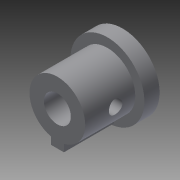
# Autodesk Inventor part: dc_to_omni_coupler_small
Saved by Autodesk Inventor 2015 (Build 190159000, 159)
## iProperties
Created: 2017-12-15
Part Number: dc_to_omni_coupler_small
Material: Generic
Document SubType Name: Modeling
Designer: Anshul
Density: 1 g/cm^3
Appearance: Default
Author: Anshul
Autodesk Inventor part; units mm, degrees
ref_plane "YZ Plane" through (0, 0, 0) normal (1, 0, 0) x (0, 1, 0)
ref_plane "XZ Plane" through (0, 0, 0) normal (0, 1, 0) x (-1, 0, 0)
sketch "Sketch1" plane through (0, 0, 0) normal (0, 1, 0) x (-1, 0, 0)
  line L0 (0, 0) -> (0, -7)
  circle A0 centre (0, -7) radius 1.55
  line L1 (3.1, 0) -> (6.4, 0)
  circle A1 centre (0, -7) radius 4
  line L2 (0, -11) -> (0, -15)
  line L3 (3.1, -15) -> (3.1, 0)
  line L4 (6.4, 0) -> (6.4, -11.5)
  line L5 (6.35, -15) -> (3.1, -15)
  line L6 (3.1, -15) -> (8.5, -15)
  line L7 (8.5, -15) -> (8.5, -11.5)
  line L8 (8.5, -11.5) -> (6.4, -11.5)
  line L9 (6.4, 0) -> (7.9, 0)
  line L10 (7.9, 0) -> (7.9, -11.5)
  line L11 (6.4, 0) -> (4.9, 0)
  line L12 (4.9, 0) -> (4.9, -11.5)
  line L13 (4.9, -11.5) -> (6.4, -11.5)
  dimension "d4" = 8
  dimension "d0" = 7
  dimension "d1" = 3.1
  dimension "d2" = 6.4
  dimension "d3" = 3.1
  dimension "d5" = 4
  dimension "d6" = 8.5
  dimension "d7" = 3.5
  dimension "d18" = 1.5
  dimension "d19" = 1.5
  constraints: 28 end point, 5 perpendicular, 3 point on line, 2 coincident, 2 horizontal, 2 parallel, 2 vertical, 1 centre point, 1 vertical alignment, 2 other
  measures "d0" distance of L0.start L0.end
  measures "d1" diameter of A0
  measures "d2" distance of L0.start L1.end
  measures "d3" distance of L1.start L0.start
  measures "d5" distance of L2.start L2.end
  measures "d6" distance of L2.end L6.end
  measures "d7" distance of L6.end L7.end
  measures "d18" distance of L1.end L9.end
  measures "d19" distance of L1.end L11.end
revolve "Revolution1" add sketch "Sketch1" angle 360 about axis through (0, 0, 0) along (0, 0, -1) picked at (3.2637, -7.5872) contours L3 L1 L12 L13 L8 L7 L6 L5 A1 | A1 L3 | L1 L4 L13 L12
ref_plane "Work Plane1" through (-6.4, 0, 0) normal (-1, 0, 0) x (0, -1, 0)
sketch "Sketch2" plane through (-6.4, 0, 0) normal (-1, 0, 0) x (0, -1, 0)
  line L0 (0, 0) -> (0, -7)
  circle A0 centre (0, -7) radius 1.55
  circle A1 centre (0, -7) radius 4
  dimension "d11" = 7
  dimension "d12" = 3.1
  dimension "d13" = 8
  constraints: 2 centre point, 2 coincident, 2 end point, 1 vertical
  measures "d11" distance of L0.start L0.end
  measures "d12" diameter of A0
  measures "d13" diameter of A1
extrude "Extrusion2" cut sketch "Sketch2" against normal blind 30 contours A0
extrude "Extrusion3" cut sketch "Sketch2" against normal blind 3
sketch "Sketch3" plane through (0, 0, 0) normal (0, 0, 1) x (1, 0, 0)
  circle A0 centre (0, 0) radius 3.1 projected
  line L0 (0, -3.1) -> (0, -6.4)
  circle A1 centre (0, 0) radius 6.4 projected
  line L1 (0, -6.4) -> (0, -7.9)
  line L2 (0, -6.4) -> (0, -4.9)
  line L3 (0, -4.9) -> (-1.5, -4.9)
  line L4 (-1.5, -4.9) -> (-1.5, -7.9)
  line L5 (-1.5, -7.9) -> (0, -7.9)
  line L6 (0, -7.9) -> (1.5, -7.9)
  line L7 (1.5, -7.9) -> (1.5, -4.9)
  line L8 (1.5, -4.9) -> (0, -4.9)
  dimension "d20" = 1.5
  dimension "d21" = 1.5
  dimension "d22" = 1.5
  dimension "d23" = 1.5
  constraints: 18 end point, 5 perpendicular, 4 point on line, 2 vertical alignment, 1 vertical, 2 other
  measures "d20" distance of L0.end L1.end
  measures "d21" distance of L0.end L2.end
  measures "d22" distance of L2.end L3.end
  measures "d23" distance of L1.end L6.end
extrude "Extrusion4" add sketch "Sketch3" against normal blind 11.5 contours L8 L7 A1 L0 | L0 A1 L4 L3 | L1 L5 L4 A1 | A1 L7 L6 L1
body "Solid1"
